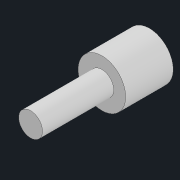
# Autodesk Inventor part: Part1
Saved by Autodesk Inventor 2022 (Build 260153000, 153)
## iProperties
Created: 2021-11-09
Part Number: Part1
Material: 一般
Document SubType Name: Modeling
Designer: Yuta Kage
Density: 1 g/cm^3
Appearance: 既定
Author: Yuta Kage
Autodesk Inventor part; units mm, degrees
ref_plane "YZ Plane" through (0, 0, 0) normal (1, 0, 0) x (0, 1, 0)
ref_plane "XZ Plane" through (0, 0, 0) normal (0, 1, 0) x (-1, 0, 0)
ref_plane "XY Plane" through (0, 0, 0) normal (0, 0, 1) x (1, 0, 0)
sketch "スケッチ1" plane through (0, 0, 0) normal (1, 0, 0) x (0, 1, 0)
  line L0 (0, 0) -> (1.5, 0)
  line L1 (1.5, 0) -> (1.5, -9)
  line L2 (1.5, -9) -> (3, -9)
  line L3 (3, -9) -> (3, -15)
  line L4 (3, -15) -> (1, -15)
  line L5 (0, 0) -> (0, -11)
  line L6 (0, -11) -> (1, -11)
  line L7 (1, -11) -> (1, -15)
  dimension "d0" = 1.5
  dimension "d1" = 1
  dimension "d2" = 9
  dimension "d3" = 4
  dimension "d4" = 2
  dimension "d5" = 2
  constraints: 17 end point, 6 perpendicular, 1 horizontal, 1 vertical
  measures "d0" distance of L0.start L0.end
  measures "d1" distance of L5.end L6.end
  measures "d2" distance of L0.end L1.end
  measures "d3" distance of L6.end L4.end
  measures "d4" distance of L3.end L4.end
  measures "d5" distance between parallel lines of L2 L6
revolve "回転1" add sketch "スケッチ1" angle 360 about axis through (0, 0, 0) along (0, 0, -1)
sketch "スケッチ2" plane through (0, 0, 0) normal (1, 0, 0) x (0, 1, 0)
  point P0 (0, 0)
  point P1 (0, -11.9211)
hole "穴1" at (0, 0, -11.9211) direction (-1, 0, 0) diameter 1.567 end through all thread size "M2x0.4" class "6H" standard "ANSI Metric M Profile"
